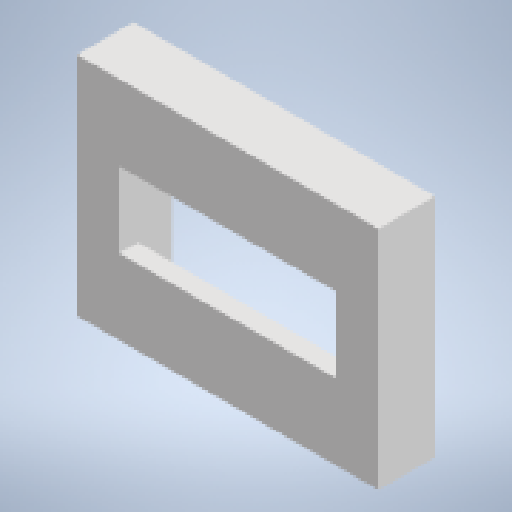
# Autodesk Inventor part: Opaque Rectangular Base
Saved by Autodesk Inventor 2024 (Build 280153000, 153)
## iProperties
Created: 2024-06-30
Part Number: Opaque Rectangular Base
Material: PET Plastic
Document SubType Name: Modeling
Designer: adam
Density: 1.541 g/cm^3
Appearance: Smooth - Black
Author: adam
Autodesk Inventor part; units mm, degrees
ref_plane "YZ Plane" through (0, 0, 0) normal (1, 0, 0) x (0, 1, 0)
ref_plane "XZ Plane" through (0, 0, 0) normal (0, 1, 0) x (-1, 0, 0)
ref_plane "XY Plane" through (0, 0, 0) normal (0, 0, 1) x (1, 0, 0)
sketch "Sketch1" plane through (0, 0, 0) normal (0, 0, 1) x (1, 0, 0)
  line L0 (-4, 3) -> (4, 3)
  line L1 (4, 3) -> (4, -3)
  line L2 (4, -3) -> (-4, -3)
  line L3 (-4, -3) -> (-4, 3)
  line L4 (-4, 3) -> (4, -3) construction
  line L5 (4, 3) -> (-4, -3) construction
  line L6 (3, 2) -> (-3, 2)
  line L7 (-3, 2) -> (-3, -2)
  line L8 (-3, -2) -> (3, -2)
  line L9 (3, -2) -> (3, 2)
  point P0 (0, 0)
  dimension "d0" = 8
  dimension "d1" = 6
  dimension "d2" = 1
  constraints: 20 end point, 4 parallel, 2 midpoint, 2 perpendicular, 1 horizontal, 3 other
  measures "d0" distance of L1.end L2.end
  measures "d1" distance of L0.end L1.end
  measures "d2" distance between parallel lines of L0 L6
extrude "Extrusion1" add sketch "Sketch1" along normal blind 1.5
sketch "Sketch2" plane through (0, 0, 1.5) normal (0, 0, 1) x (1, 0, 0)
  line L0 (4, 3) -> (-4, 3) projected
  line L1 (-4, -3) -> (4, -3) projected
  line L2 (-4, 3) -> (4, 3)
  line L3 (4, 3) -> (4, -3)
  line L4 (4, -3) -> (-4, -3)
  line L5 (-4, -3) -> (-4, 3)
  line L6 (-3, 1.125) -> (3, 1.125)
  line L7 (3, 1.125) -> (3, -1.125)
  line L8 (3, -1.125) -> (-3, -1.125)
  line L9 (-3, -1.125) -> (-3, 1.125)
  line L10 (-3, 1.125) -> (3, -1.125) construction
  line L11 (3, 1.125) -> (-3, -1.125) construction
  point P0 (0, 0)
  dimension "d5" = 6
  dimension "d6" = 2.25
  constraints: 20 end point, 4 parallel, 2 horizontal, 2 midpoint, 2 perpendicular
  measures "d5" distance of L7.end L8.end
  measures "d6" distance of L6.end L7.end
extrude "Extrusion2" add sketch "Sketch2" along normal blind 0.5
body "Solid1"
